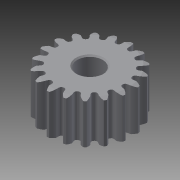
# Autodesk Inventor part: GEAHB1.0-18-10-A-6_b
Saved by Autodesk Inventor 2014 SP2 (Build 180246200, 246)
## iProperties
Created: 2019-03-13
Part Number: GEAHB1.0-18-10-A-6_b
Material: Generic
Catalog Web Link: www.cadenas.de
Description: GEAHB1.0, GEAHBB1.0, GEAHBG1.0, GEAHS1.0, GEAB1.0, GEABB1.0, GEABG1.0, GEAS1.0, GEAKB1.0, GEAKBB1.0, GEAKBG1.0, GEAKS1.0_body-Spur Gears - Pressure Angle 20 Degree Module 1.0
Vendor: MISUMI
Document SubType Name: Modeling
Designer: psadmin
Manufacturer: MISUMI
Mass: 2.186 g
Surface Area: 17.0541 cm^2
Volume: 2.186 cm^3
Density: 1 g/cm^3
Appearance: PSOLRGB-192-192-192
Category: PARTsolutions
Company: MISUMI
Title: GEAHB1.0-18-10-A-6
Author: Cadenas PARTsolutions
Comments: Spur Gears - Pressure Angle 20 Degree Module 1.0
PSOL_IDENT_0: {$CADENAS_DATA\23d-libs\misumi\metric\54_spur_gears\geab10\geab10.prj},526 {VTYP=3D},{NB=GEAHB1.0-18
PSOL_IDENT_1: -10-A-6_b},{LINA=GEAHB1.0-18-10-A-6},{NN=GEAHB1.0, GEAHBB1.0, GEAHBG1.0, GEAHS1.0, GEAB1.0, GEABB1.0
PSOL_IDENT_2: , GEABG1.0, GEAS1.0, GEAKB1.0, GEAKBB1.0, GEAKBG1.0, GEAKS1.0_body},{DATE=12.06.2018 01:08:09},{GEOM
PSOL_IDENT_3: DATE=12.06.2018 01:08:00},{VERSION=},{LINEID=20},{WBVAR=SHS,MAT,ST,NT,B,TSSE,TS,PS,ALT1,ALT2,TPC,ALT
PSOL_IDENT_4: 11,ALT10,BS,ALT4,Z,J,ALT5,Q,R,S,T,ALT9,SRG,ALT6,LFC,LTC,MALT6,ALT7,KFC,KTC,K,ALT3,DIRALT3,QFC,QTC,MA
PSOL_IDENT_5: LT3,ALT8,DIRALT8,ZFC,ZTC,U},{WBNUMERIC=NT,B,BS,Z,J,Q,R,S,T,SRG,LFC,LTC,KFC,KTC,K,QFC,QTC,ZFC,ZTC,U}
PSOL_IDENT_6: {NB=GEAHB1.0-18-10-A-6_b},{LINA=GEAHB1.0-18-10-A-6},{KT=DUMMY},{PN=GEAHB1.0-18-10-A-6},{SHS=RH},{TY
PSOL_IDENT_7: PE=GEAHB},{MAT=S45C},{MATALG= 'S45C','S45C Equivalent','SUS304','SUS304' },{ST=},{STALG= '','-','BO'
PSOL_IDENT_8: ,'Black Oxide','ENP','Electroless Nickel Plating'},{AC=-},{MOD=1.0},{NT=18},{NTALG=12,13,14,15,16,17
PSOL_IDENT_9: ,18,19,20,21,22,23,24,25,26,27,28,29,30,32,33,34,35,36,38,39,40,42,44,45,46,48,49,50,51,52,54,55,56,
PSOL_IDENT_10: 57,58,60,62,63,64,65,66,68,69,70,72,75,76,77,78,80,81,84,85,88,90,91,92,95,96,98,99,100,110,120},{B=
PSOL_IDENT_11: 10},{BALG=6,8,10,12},{TSSE=TSSE},{TSSEALG= '','Not Specified','TSSE','Specified'},{TS=A},{TSALG='K','
PSOL_IDENT_12: K','A','A'},{TSPN=-A},{PS=6},{PSALG='6','6','6.35','6.35','7','7','8','8','9','9','10','10','11','11'
PSOL_IDENT_13: ,'12','12'},{P=6.00},{DD=18},{D=20},{G=15.5},{H=0},{L=0},{LL1=0},{LL2=0},{M=-},{ML=0.000},{ALT1=},{A
PSOL_IDENT_14: LT1ALG= '','N/A' },{ALT1PN=},{KC=0},{ALT2=},{ALT2ALG= '','N/A' },{TPC=N/A},{TPCALG= 'N/A' },{ALT2PN=
PSOL_IDENT_15: },{ALT11=},{ALT11ALG= '','N/A' },{ALT11PN=},{DEG=0},{ALT10=},{ALT10ALG= '','Not applicable' },{BS=0.
PSOL_IDENT_16: 0},{BSALG=0},{BSMIN=3},{BSMAX=0},{ALT10PN=},{LL13D=0},{LL23D=0},{LBS=10},{ALT4=},{ALT4ALG='','w/o St
PSOL_IDENT_17: epped Hole','DHL','with DHL (Stepped Hole)','DHR','with DHR (Stepped Hole)'},{ALT41=1},{ALT42=1},{AL
PSOL_IDENT_18: T4PN=},{Z=0},{ZALG=0},{ZPN=},{ZMINL=8},{ZMAXL=11},{ZMINR=8},{ZMAXR=11},{J=0.0},{JALG=0},{JPN=},{JMIN=
PSOL_IDENT_19: 2.0},{JMAX=0.0},{ALT5=},{ALT5ALG= '','w/o WDH (Both Ends Stepped Hole)','WDH','with WDH (Both Ends S
PSOL_IDENT_20: tepped Hole)' },{ALT5PN=},{Q=0},{QALG=0},{QPN=},{QMIN=8},{QMAX=11},{R=0},{RALG=0},{RPN=},{RMIN=8},{R
PSOL_IDENT_21: MAX=11.0},{S=0},{SALG=0},{SPN=},{SMIN=3},{SMAX=4},{T=0},{TALG=0},{TPN=},{TMIN=3},{TMAX=0},{ALT9=},{A
PSOL_IDENT_22: LT9ALG= '','Not applicable' },{SRG=0.0},{SRGALG=0},{SRGMIN=3.500},{SRGMINALG=3.500},{SRGMAX=0.000},{
PSOL_IDENT_23: SRGMAXALG=0.000},{DD2=0.0},{MM=0.00},{NN=0.00},{DD2ALG=0.000},{MMALG=0.000},{NNALG=0.000},{ALT9PN=},
PSOL_IDENT_24: {ALT6=},{ALT6ALG= '','Not applicable' },{ALT6PN=},{LFC=0},{LFCALG=0},{LTC=0},{LTCALG=0},{LPCDMIN=14}
PSOL_IDENT_25: ,{LPCDMAX=8},{MALT6=N/A},{MALT6ALG= 'N/A' },{C=0.0},{ALT7=},{ALT7ALG= '','Not applicable' },{ALT7PN=
PSOL_IDENT_26: },{KFC=0},{KFCALG=[0]},{KTC=0},{KTCALG=[0]},{KPCDMIN1=13},{KPCDMAX1=-7},{KPCDMIN2=7},{KPCDMAX2=8},{K
PSOL_IDENT_27: PCD=0},{K=0.0},{KALG=[0]},{KALT7L=10},{SCREW=0},{SCREWL=0},{ALT3=},{ALT3ALG= '','Not applicable' },{
PSOL_IDENT_28: DIRALT3=},{DIRALT3ALG= '','N/A' },{ALT3PN=},{QFC=0},{QFCALG=[0]},{QTC=0},{QTCALG=[0]},{QPCDMIN1=13},
PSOL_IDENT_29: {QPCDMAX1=-7},{QPCDMIN2=7},{QPCDMAX2=8},{CIFMALT3=3},{QPCD=0},{MALT3=N/A},{MALT3ALG= 'N/A' },{MALT3L=
PSOL_IDENT_30: 0},{MS1=3},{PITCH=0},{BB=0},{TT=0},{ALT8=},{ALT8ALG= '','Not applicable' },{DIRALT8=},{DIRALT8ALG= ''
PSOL_IDENT_31: ,'N/A' },{ALT8PN=},{ZFC=0},{ZFCALG=[0]},{ZFCMIN=16},{ZFCMAX=5},{ZTC=0},{ZTCALG=[0]},{ZPCDMIN1=16},{Z
PSOL_IDENT_32: PCDMIN2=11},{ZPCDMAX1=-10},{ZPCDMAX2=5},{ZPCD=0},{U=0},{UALG=[0]},{UMAX=0},{UMAX1=0},{UMAX2=4},{UMIN=
PSOL_IDENT_33: 3},{U1=0.0},{U2=0.0},{F=0.0},{PLANE=3},{BL1=10},{BL2=9.5},{PCD=0},{SHN=0},{SHDEG1=0},{SHDEG2=0},{PZQ
PSOL_IDENT_34: RDD2=6},{ALT3LBS=9.5},{D1=5},{D2=10},{D3=20},{D4=0.1},{D5=3},{D6=2.769231},{D7=0.85},{D8=0.5},{D9=0.
PSOL_IDENT_35: 812072},{S1=15},{S2=1},{KR=22.5}
NN: 0
NT: 18
NB: GEAHB1.0-18-10-A-6_b
NBSYN: $PN._b
LINA: GEAHB1.0-18-10-A-6
PN: GEAHB1.0-18-10-A-6
SHS: Round Hole
MAT: S45C Equivalent
ST: -
AC: -
MOD: 1
B: 10
TSSE: Specified
TS: A
PS: 6
DD: 18
D: 20
G: 15.5
H: 0
L: 0
LL1: 0
LL2: 0
M: -
ALT1: N/A
ALT2: N/A
TPC: N/A
ALT11: N/A
ALT10: Not applicable
BS: 0
ALT4: w/o Stepped Hole
Z: 0
J: 0
ALT5: w/o WDH (Both Ends Stepped Hole)
Q: 0
R: 0
S: 0
T: 0
ALT9: Not applicable
SRG: 0
DD2: 0
MM: 0
ALT6: Not applicable
LFC: 0
LTC: 0
MALT6: N/A
C: 0
ALT7: Not applicable
KFC: 0
KTC: 0
K: 0
ALT3: Not applicable
DIRALT3: N/A
QFC: 0
QTC: 0
MALT3: N/A
ALT8: Not applicable
DIRALT8: N/A
ZFC: 0
ZTC: 0
U: 0
U1: 0
U2: 0
F: 0
SUPPLIER: MISUMI
ARTICLENO: GEAHB1.0-18-10-A-6_b
BOMINFO: GEAHB1.0-18-10-A-6
CREATOR: CADENAS GmbH
Autodesk Inventor part; units mm, degrees
sketch "Sketch_12" plane through (0, 0, 0) normal (1, 0, 0) x (0, 1, 0)
  line L0 (0, 0) -> (0, 10)
  line L1 (0, 10) -> (9, 10)
  line L2 (9, 10) -> (15, 8.3923)
  line L3 (15, 8.3923) -> (15, 1.6077)
  line L4 (15, 1.6077) -> (9, 0)
  line L5 (9, 0) -> (0, 0)
  line L6 (0, 0) -> (0, 10)
  constraints: 14 end point
revolve "Revolution1" add sketch "Sketch_12" angle 360 about axis through (0, 0, 0) along (0, 0, -1)
sketch "Sketch_3" plane through (0, 0, 0) normal (0, 0, 1) x (1, 0, 0)
  circle A0 centre (0, 0) radius 40
  arc A1 (-9.8858, 1.507) -> (-9.859, 1.4225) centre (-9.7869, 1.4919) ccw
  arc A2 (-9.859, 1.4225) -> (-8.9658, 0.7844) centre (-7.6979, 3.5033) ccw
  arc A3 (-8.9658, 0.7844) -> (-8.707, 0.7127) centre (-8.6226, 1.5204) ccw
  arc A4 (-8.0844, 0.573) -> (-8.707, 0.7127) centre (-8.9979, -2.0412) ccw
  arc A5 (-7.7494, 0.0949) -> (-8.0844, 0.573) centre (-8.2494, 0.101) ccw
  arc A6 (-7.7494, 0.0949) -> (-7.7494, -0.0949) centre (0, 0) ccw
  arc A7 (-8.0844, -0.573) -> (-7.7494, -0.0949) centre (-8.2494, -0.101) ccw
  arc A8 (-8.707, -0.7127) -> (-8.0844, -0.573) centre (-8.9979, 2.0412) ccw
  arc A9 (-8.707, -0.7127) -> (-8.9658, -0.7844) centre (-8.6226, -1.5204) ccw
  arc A10 (-8.9658, -0.7844) -> (-9.859, -1.4225) centre (-7.6979, -3.5033) ccw
  arc A11 (-9.859, -1.4225) -> (-9.8858, -1.507) centre (-9.7869, -1.4919) ccw
  arc A12 (-9.8858, -1.507) -> (-9.805, -1.9651) centre (0, 0) ccw
  arc A13 (-9.805, -1.9651) -> (-9.7509, -2.0352) centre (-9.707, -1.9454) ccw
  arc A14 (-9.7509, -2.0352) -> (-8.6933, -2.3294) centre (-8.4319, 0.6592) ccw
  arc A15 (-8.6933, -2.3294) -> (-8.4257, -2.3082) centre (-8.6226, -1.5204) ccw
  arc A16 (-7.7929, -2.2266) -> (-8.4257, -2.3082) centre (-7.7572, -4.9956) ccw
  arc A17 (-7.3145, -2.5613) -> (-7.7929, -2.2266) centre (-7.7864, -2.7265) ccw
  arc A18 (-7.3145, -2.5613) -> (-7.2496, -2.7396) centre (0, 0) ccw
  arc A19 (-7.4009, -3.3035) -> (-7.2496, -2.7396) centre (-7.7173, -2.9164) ccw
  arc A20 (-7.9381, -3.6477) -> (-7.4009, -3.3035) centre (-9.1534, -1.1594) ccw
  arc A21 (-7.9381, -3.6477) -> (-8.1568, -3.8036) centre (-7.5825, -4.3778) ccw
  arc A22 (-8.1568, -3.8036) -> (-8.7779, -4.7087) centre (-6.0354, -5.9249) ccw
  arc A23 (-8.7779, -4.7087) -> (-8.7742, -4.7972) centre (-8.6865, -4.7492) ccw
  arc A24 (-8.7742, -4.7972) -> (-8.5416, -5.2001) centre (0, 0) ccw
  arc A25 (-8.5416, -5.2001) -> (-8.4668, -5.2475) centre (-8.4562, -5.1481) ccw
  arc A26 (-8.4668, -5.2475) -> (-7.3724, -5.1622) centre (-8.1488, -2.2644) ccw
  arc A27 (-7.3724, -5.1622) -> (-7.1281, -5.0508) centre (-7.5825, -4.3778) ccw
  arc A28 (-6.5614, -4.7576) -> (-7.1281, -5.0508) centre (-5.5808, -7.3474) ccw
  arc A29 (-5.9974, -4.9085) -> (-6.5614, -4.7576) centre (-6.3843, -5.2252) ccw
  arc A30 (-5.9974, -4.9085) -> (-5.8754, -5.0539) centre (0, 0) ccw
  arc A31 (-5.8247, -5.6356) -> (-5.8754, -5.0539) centre (-6.2545, -5.38) ccw
  arc A32 (-6.2118, -6.1427) -> (-5.8247, -5.6356) centre (-8.2049, -4.2201) ccw
  arc A33 (-6.2118, -6.1427) -> (-6.364, -6.364) centre (-5.628, -6.7072) ccw
  arc A34 (-6.364, -6.364) -> (-6.638, -7.4269) centre (-3.645, -7.6318) ccw
  arc A35 (-6.638, -7.4269) -> (-6.6043, -7.5089) centre (-6.5383, -7.4338) ccw
  arc A36 (-6.6043, -7.5089) -> (-6.248, -7.8079) centre (0, 0) ccw
  arc A37 (-6.248, -7.8079) -> (-6.1614, -7.8269) centre (-6.1855, -7.7298) ccw
  arc A38 (-6.1614, -7.8269) -> (-5.1622, -7.3724) centre (-6.8829, -4.9149) ccw
  arc A39 (-5.1622, -7.3724) -> (-4.9707, -7.1841) centre (-5.628, -6.7072) ccw
  arc A40 (-4.5385, -6.7148) -> (-4.9707, -7.1841) centre (-2.7312, -8.813) ccw
  arc A41 (-3.9569, -6.6637) -> (-4.5385, -6.7148) centre (-4.2122, -7.0937) ccw
  arc A42 (-3.9569, -6.6637) -> (-3.7925, -6.7586) centre (0, 0) ccw
  arc A43 (-3.546, -7.2879) -> (-3.7925, -6.7586) centre (-4.0372, -7.1947) ccw
  arc A44 (-3.7363, -7.8968) -> (-3.546, -7.2879) centre (-6.2667, -6.7718) ccw
  arc A45 (-3.7363, -7.8968) -> (-3.8036, -8.1568) centre (-2.9946, -8.2275) ccw
  arc A46 (-3.8036, -8.1568) -> (-3.6975, -9.2494) centre (-0.815, -8.4182) ccw
  arc A47 (-3.6975, -9.2494) -> (-3.6378, -9.3148) centre (-3.6015, -9.2217) ccw
  arc A48 (-3.6378, -9.3148) -> (-3.2007, -9.4739) centre (0, 0) ccw
  arc A49 (-3.2007, -9.4739) -> (-3.1129, -9.4622) centre (-3.1687, -9.3792) ccw
  arc A50 (-3.1129, -9.4622) -> (-2.3294, -8.6933) centre (-4.7868, -6.9726) ccw
  arc A51 (-2.3294, -8.6933) -> (-2.2138, -8.4509) centre (-2.9946, -8.2275) ccw
  arc A52 (-1.9682, -7.8621) -> (-2.2138, -8.4509) centre (0.4477, -9.2157) ccw
  arc A53 (-1.4391, -7.6152) -> (-1.9682, -7.8621) centre (-1.532, -8.1065) ccw
  arc A54 (-1.4391, -7.6152) -> (-1.2522, -7.6482) centre (0, 0) ccw
  arc A55 (-0.8395, -8.0611) -> (-1.2522, -7.6482) centre (-1.333, -8.1416) ccw
  arc A56 (-0.8101, -8.6985) -> (-0.8395, -8.0611) centre (-3.5727, -8.5068) ccw
  arc A57 (-0.8101, -8.6985) -> (-0.7844, -8.9658) centre (0, -8.7556) ccw
  arc A58 (-0.7844, -8.9658) -> (-0.3111, -9.9562) centre (2.1134, -8.1893) ccw
  arc A59 (-0.3111, -9.9562) -> (-0.2326, -9.9973) centre (-0.2303, -9.8973) ccw
  arc A60 (-0.2326, -9.9973) -> (0.2326, -9.9973) centre (0, 0) ccw
  arc A61 (0.2326, -9.9973) -> (0.3111, -9.9562) centre (0.2303, -9.8973) ccw
  arc A62 (0.3111, -9.9562) -> (0.7844, -8.9658) centre (-2.1134, -8.1893) ccw
  arc A63 (0.7844, -8.9658) -> (0.8101, -8.6985) centre (0, -8.7556) ccw
  arc A64 (0.8395, -8.0611) -> (0.8101, -8.6985) centre (3.5727, -8.5068) ccw
  arc A65 (1.2522, -7.6482) -> (0.8395, -8.0611) centre (1.333, -8.1416) ccw
  arc A66 (1.2522, -7.6482) -> (1.4391, -7.6152) centre (0, 0) ccw
  arc A67 (1.9682, -7.8621) -> (1.4391, -7.6152) centre (1.532, -8.1065) ccw
  arc A68 (2.2138, -8.4509) -> (1.9682, -7.8621) centre (-0.4477, -9.2157) ccw
  arc A69 (2.2138, -8.4509) -> (2.3294, -8.6933) centre (2.9946, -8.2275) ccw
  arc A70 (2.3294, -8.6933) -> (3.1129, -9.4622) centre (4.7868, -6.9726) ccw
  arc A71 (3.1129, -9.4622) -> (3.2007, -9.4739) centre (3.1687, -9.3792) ccw
  arc A72 (3.2007, -9.4739) -> (3.6378, -9.3148) centre (0, 0) ccw
  arc A73 (3.6378, -9.3148) -> (3.6975, -9.2494) centre (3.6015, -9.2217) ccw
  arc A74 (3.6975, -9.2494) -> (3.8036, -8.1568) centre (0.815, -8.4182) ccw
  arc A75 (3.8036, -8.1568) -> (3.7363, -7.8968) centre (2.9946, -8.2275) ccw
  arc A76 (3.546, -7.2879) -> (3.7363, -7.8968) centre (6.2667, -6.7718) ccw
  arc A77 (3.7925, -6.7586) -> (3.546, -7.2879) centre (4.0372, -7.1947) ccw
  arc A78 (3.7925, -6.7586) -> (3.9569, -6.6637) centre (0, 0) ccw
  arc A79 (4.5385, -6.7148) -> (3.9569, -6.6637) centre (4.2122, -7.0937) ccw
  arc A80 (4.9707, -7.1841) -> (4.5385, -6.7148) centre (2.7312, -8.813) ccw
  arc A81 (4.9707, -7.1841) -> (5.1622, -7.3724) centre (5.628, -6.7072) ccw
  arc A82 (5.1622, -7.3724) -> (6.1614, -7.8269) centre (6.8829, -4.9149) ccw
  arc A83 (6.1614, -7.8269) -> (6.248, -7.8079) centre (6.1855, -7.7298) ccw
  arc A84 (6.248, -7.8079) -> (6.6043, -7.5089) centre (0, 0) ccw
  arc A85 (6.6043, -7.5089) -> (6.638, -7.4269) centre (6.5383, -7.4338) ccw
  arc A86 (6.638, -7.4269) -> (6.364, -6.364) centre (3.645, -7.6318) ccw
  arc A87 (6.364, -6.364) -> (6.2118, -6.1427) centre (5.628, -6.7072) ccw
  arc A88 (5.8247, -5.6356) -> (6.2118, -6.1427) centre (8.2049, -4.2201) ccw
  arc A89 (5.8754, -5.0539) -> (5.8247, -5.6356) centre (6.2545, -5.38) ccw
  arc A90 (5.8754, -5.0539) -> (5.9974, -4.9085) centre (0, 0) ccw
  arc A91 (6.5614, -4.7576) -> (5.9974, -4.9085) centre (6.3843, -5.2252) ccw
  arc A92 (7.1281, -5.0508) -> (6.5614, -4.7576) centre (5.5808, -7.3474) ccw
  arc A93 (7.1281, -5.0508) -> (7.3724, -5.1622) centre (7.5825, -4.3778) ccw
  arc A94 (7.3724, -5.1622) -> (8.4668, -5.2475) centre (8.1488, -2.2644) ccw
  arc A95 (8.4668, -5.2475) -> (8.5416, -5.2001) centre (8.4562, -5.1481) ccw
  arc A96 (8.5416, -5.2001) -> (8.7742, -4.7972) centre (0, 0) ccw
  arc A97 (8.7742, -4.7972) -> (8.7779, -4.7087) centre (8.6865, -4.7492) ccw
  arc A98 (8.7779, -4.7087) -> (8.1568, -3.8036) centre (6.0354, -5.9249) ccw
  arc A99 (8.1568, -3.8036) -> (7.9381, -3.6477) centre (7.5825, -4.3778) ccw
  arc A100 (7.4009, -3.3035) -> (7.9381, -3.6477) centre (9.1534, -1.1594) ccw
  arc A101 (7.2496, -2.7396) -> (7.4009, -3.3035) centre (7.7173, -2.9164) ccw
  arc A102 (7.2496, -2.7396) -> (7.3145, -2.5613) centre (0, 0) ccw
  arc A103 (7.7929, -2.2266) -> (7.3145, -2.5613) centre (7.7864, -2.7265) ccw
  arc A104 (8.4257, -2.3082) -> (7.7929, -2.2266) centre (7.7572, -4.9956) ccw
  arc A105 (8.4257, -2.3082) -> (8.6933, -2.3294) centre (8.6226, -1.5204) ccw
  arc A106 (8.6933, -2.3294) -> (9.7509, -2.0352) centre (8.4319, 0.6592) ccw
  arc A107 (9.7509, -2.0352) -> (9.805, -1.9651) centre (9.707, -1.9454) ccw
  arc A108 (9.805, -1.9651) -> (9.8858, -1.507) centre (0, 0) ccw
  arc A109 (9.8858, -1.507) -> (9.859, -1.4225) centre (9.7869, -1.4919) ccw
  arc A110 (9.859, -1.4225) -> (8.9658, -0.7844) centre (7.6979, -3.5033) ccw
  arc A111 (8.9658, -0.7844) -> (8.707, -0.7127) centre (8.6226, -1.5204) ccw
  arc A112 (8.0844, -0.573) -> (8.707, -0.7127) centre (8.9979, 2.0412) ccw
  arc A113 (7.7494, -0.0949) -> (8.0844, -0.573) centre (8.2494, -0.101) ccw
  arc A114 (7.7494, -0.0949) -> (7.7494, 0.0949) centre (0, 0) ccw
  arc A115 (8.0844, 0.573) -> (7.7494, 0.0949) centre (8.2494, 0.101) ccw
  arc A116 (8.707, 0.7127) -> (8.0844, 0.573) centre (8.9979, -2.0412) ccw
  arc A117 (8.707, 0.7127) -> (8.9658, 0.7844) centre (8.6226, 1.5204) ccw
  arc A118 (8.9658, 0.7844) -> (9.859, 1.4225) centre (7.6979, 3.5033) ccw
  arc A119 (9.859, 1.4225) -> (9.8858, 1.507) centre (9.7869, 1.4919) ccw
  arc A120 (9.8858, 1.507) -> (9.805, 1.9651) centre (0, 0) ccw
  arc A121 (9.805, 1.9651) -> (9.7509, 2.0352) centre (9.707, 1.9454) ccw
  arc A122 (9.7509, 2.0352) -> (8.6933, 2.3294) centre (8.4319, -0.6592) ccw
  arc A123 (8.6933, 2.3294) -> (8.4257, 2.3082) centre (8.6226, 1.5204) ccw
  arc A124 (7.7929, 2.2266) -> (8.4257, 2.3082) centre (7.7572, 4.9956) ccw
  arc A125 (7.3145, 2.5613) -> (7.7929, 2.2266) centre (7.7864, 2.7265) ccw
  arc A126 (7.3145, 2.5613) -> (7.2496, 2.7396) centre (0, 0) ccw
  arc A127 (7.4009, 3.3035) -> (7.2496, 2.7396) centre (7.7173, 2.9164) ccw
  arc A128 (7.9381, 3.6477) -> (7.4009, 3.3035) centre (9.1534, 1.1594) ccw
  arc A129 (7.9381, 3.6477) -> (8.1568, 3.8036) centre (7.5825, 4.3778) ccw
  arc A130 (8.1568, 3.8036) -> (8.7779, 4.7087) centre (6.0354, 5.9249) ccw
  arc A131 (8.7779, 4.7087) -> (8.7742, 4.7972) centre (8.6865, 4.7492) ccw
  arc A132 (8.7742, 4.7972) -> (8.5416, 5.2001) centre (0, 0) ccw
  arc A133 (8.5416, 5.2001) -> (8.4668, 5.2475) centre (8.4562, 5.1481) ccw
  arc A134 (8.4668, 5.2475) -> (7.3724, 5.1622) centre (8.1488, 2.2644) ccw
  arc A135 (7.3724, 5.1622) -> (7.1281, 5.0508) centre (7.5825, 4.3778) ccw
  arc A136 (6.5614, 4.7576) -> (7.1281, 5.0508) centre (5.5808, 7.3474) ccw
  arc A137 (5.9974, 4.9085) -> (6.5614, 4.7576) centre (6.3843, 5.2252) ccw
  arc A138 (5.9974, 4.9085) -> (5.8754, 5.0539) centre (0, 0) ccw
  arc A139 (5.8247, 5.6356) -> (5.8754, 5.0539) centre (6.2545, 5.38) ccw
  arc A140 (6.2118, 6.1427) -> (5.8247, 5.6356) centre (8.2049, 4.2201) ccw
  arc A141 (6.2118, 6.1427) -> (6.364, 6.364) centre (5.628, 6.7072) ccw
  arc A142 (6.364, 6.364) -> (6.638, 7.4269) centre (3.645, 7.6318) ccw
  arc A143 (6.638, 7.4269) -> (6.6043, 7.5089) centre (6.5383, 7.4338) ccw
  arc A144 (6.6043, 7.5089) -> (6.248, 7.8079) centre (0, 0) ccw
  arc A145 (6.248, 7.8079) -> (6.1614, 7.8269) centre (6.1855, 7.7298) ccw
  arc A146 (6.1614, 7.8269) -> (5.1622, 7.3724) centre (6.8829, 4.9149) ccw
  arc A147 (5.1622, 7.3724) -> (4.9707, 7.1841) centre (5.628, 6.7072) ccw
  arc A148 (4.5385, 6.7148) -> (4.9707, 7.1841) centre (2.7312, 8.813) ccw
  arc A149 (3.9569, 6.6637) -> (4.5385, 6.7148) centre (4.2122, 7.0937) ccw
  arc A150 (3.9569, 6.6637) -> (3.7925, 6.7586) centre (0, 0) ccw
  arc A151 (3.546, 7.2879) -> (3.7925, 6.7586) centre (4.0372, 7.1947) ccw
  arc A152 (3.7363, 7.8968) -> (3.546, 7.2879) centre (6.2667, 6.7718) ccw
  arc A153 (3.7363, 7.8968) -> (3.8036, 8.1568) centre (2.9946, 8.2275) ccw
  arc A154 (3.8036, 8.1568) -> (3.6975, 9.2494) centre (0.815, 8.4182) ccw
  arc A155 (3.6975, 9.2494) -> (3.6378, 9.3148) centre (3.6015, 9.2217) ccw
  arc A156 (3.6378, 9.3148) -> (3.2007, 9.4739) centre (0, 0) ccw
  arc A157 (3.2007, 9.4739) -> (3.1129, 9.4622) centre (3.1687, 9.3792) ccw
  arc A158 (3.1129, 9.4622) -> (2.3294, 8.6933) centre (4.7868, 6.9726) ccw
  arc A159 (2.3294, 8.6933) -> (2.2138, 8.4509) centre (2.9946, 8.2275) ccw
  arc A160 (1.9682, 7.8621) -> (2.2138, 8.4509) centre (-0.4477, 9.2157) ccw
  arc A161 (1.4391, 7.6152) -> (1.9682, 7.8621) centre (1.532, 8.1065) ccw
  arc A162 (1.4391, 7.6152) -> (1.2522, 7.6482) centre (0, 0) ccw
  arc A163 (0.8395, 8.0611) -> (1.2522, 7.6482) centre (1.333, 8.1416) ccw
  arc A164 (0.8101, 8.6985) -> (0.8395, 8.0611) centre (3.5727, 8.5068) ccw
  arc A165 (0.8101, 8.6985) -> (0.7844, 8.9658) centre (0, 8.7556) ccw
  arc A166 (0.7844, 8.9658) -> (0.3111, 9.9562) centre (-2.1134, 8.1893) ccw
  arc A167 (0.3111, 9.9562) -> (0.2326, 9.9973) centre (0.2303, 9.8973) ccw
  arc A168 (0.2326, 9.9973) -> (-0.2326, 9.9973) centre (0, 0) ccw
  arc A169 (-0.2326, 9.9973) -> (-0.3111, 9.9562) centre (-0.2303, 9.8973) ccw
  arc A170 (-0.3111, 9.9562) -> (-0.7844, 8.9658) centre (2.1134, 8.1893) ccw
  arc A171 (-0.7844, 8.9658) -> (-0.8101, 8.6985) centre (0, 8.7556) ccw
  arc A172 (-0.8395, 8.0611) -> (-0.8101, 8.6985) centre (-3.5727, 8.5068) ccw
  arc A173 (-1.2522, 7.6482) -> (-0.8395, 8.0611) centre (-1.333, 8.1416) ccw
  arc A174 (-1.2522, 7.6482) -> (-1.4391, 7.6152) centre (0, 0) ccw
  arc A175 (-1.9682, 7.8621) -> (-1.4391, 7.6152) centre (-1.532, 8.1065) ccw
  arc A176 (-2.2138, 8.4509) -> (-1.9682, 7.8621) centre (0.4477, 9.2157) ccw
  arc A177 (-2.2138, 8.4509) -> (-2.3294, 8.6933) centre (-2.9946, 8.2275) ccw
  arc A178 (-2.3294, 8.6933) -> (-3.1129, 9.4622) centre (-4.7868, 6.9726) ccw
  arc A179 (-3.1129, 9.4622) -> (-3.2007, 9.4739) centre (-3.1687, 9.3792) ccw
  arc A180 (-3.2007, 9.4739) -> (-3.6378, 9.3148) centre (0, 0) ccw
  arc A181 (-3.6378, 9.3148) -> (-3.6975, 9.2494) centre (-3.6015, 9.2217) ccw
  arc A182 (-3.6975, 9.2494) -> (-3.8036, 8.1568) centre (-0.815, 8.4182) ccw
  arc A183 (-3.8036, 8.1568) -> (-3.7363, 7.8968) centre (-2.9946, 8.2275) ccw
  arc A184 (-3.546, 7.2879) -> (-3.7363, 7.8968) centre (-6.2667, 6.7718) ccw
  arc A185 (-3.7925, 6.7586) -> (-3.546, 7.2879) centre (-4.0372, 7.1947) ccw
  arc A186 (-3.7925, 6.7586) -> (-3.9569, 6.6637) centre (0, 0) ccw
  arc A187 (-4.5385, 6.7148) -> (-3.9569, 6.6637) centre (-4.2122, 7.0937) ccw
  arc A188 (-4.9707, 7.1841) -> (-4.5385, 6.7148) centre (-2.7312, 8.813) ccw
  arc A189 (-4.9707, 7.1841) -> (-5.1622, 7.3724) centre (-5.628, 6.7072) ccw
  arc A190 (-5.1622, 7.3724) -> (-6.1614, 7.8269) centre (-6.8829, 4.9149) ccw
  arc A191 (-6.1614, 7.8269) -> (-6.248, 7.8079) centre (-6.1855, 7.7298) ccw
  arc A192 (-6.248, 7.8079) -> (-6.6043, 7.5089) centre (0, 0) ccw
  arc A193 (-6.6043, 7.5089) -> (-6.638, 7.4269) centre (-6.5383, 7.4338) ccw
  arc A194 (-6.638, 7.4269) -> (-6.364, 6.364) centre (-3.645, 7.6318) ccw
  arc A195 (-6.364, 6.364) -> (-6.2118, 6.1427) centre (-5.628, 6.7072) ccw
  arc A196 (-5.8247, 5.6356) -> (-6.2118, 6.1427) centre (-8.2049, 4.2201) ccw
  arc A197 (-5.8754, 5.0539) -> (-5.8247, 5.6356) centre (-6.2545, 5.38) ccw
  arc A198 (-5.8754, 5.0539) -> (-5.9974, 4.9085) centre (0, 0) ccw
  arc A199 (-6.5614, 4.7576) -> (-5.9974, 4.9085) centre (-6.3843, 5.2252) ccw
  arc A200 (-7.1281, 5.0508) -> (-6.5614, 4.7576) centre (-5.5808, 7.3474) ccw
  arc A201 (-7.1281, 5.0508) -> (-7.3724, 5.1622) centre (-7.5825, 4.3778) ccw
  arc A202 (-7.3724, 5.1622) -> (-8.4668, 5.2475) centre (-8.1488, 2.2644) ccw
  arc A203 (-8.4668, 5.2475) -> (-8.5416, 5.2001) centre (-8.4562, 5.1481) ccw
  arc A204 (-8.5416, 5.2001) -> (-8.7742, 4.7972) centre (0, 0) ccw
  arc A205 (-8.7742, 4.7972) -> (-8.7779, 4.7087) centre (-8.6865, 4.7492) ccw
  arc A206 (-8.7779, 4.7087) -> (-8.1568, 3.8036) centre (-6.0354, 5.9249) ccw
  arc A207 (-8.1568, 3.8036) -> (-7.9381, 3.6477) centre (-7.5825, 4.3778) ccw
  arc A208 (-7.4009, 3.3035) -> (-7.9381, 3.6477) centre (-9.1534, 1.1594) ccw
  arc A209 (-7.2496, 2.7396) -> (-7.4009, 3.3035) centre (-7.7173, 2.9164) ccw
  arc A210 (-7.2496, 2.7396) -> (-7.3145, 2.5613) centre (0, 0) ccw
  arc A211 (-7.7929, 2.2266) -> (-7.3145, 2.5613) centre (-7.7864, 2.7265) ccw
  arc A212 (-8.4257, 2.3082) -> (-7.7929, 2.2266) centre (-7.7572, 4.9956) ccw
  arc A213 (-8.4257, 2.3082) -> (-8.6933, 2.3294) centre (-8.6226, 1.5204) ccw
  arc A214 (-8.6933, 2.3294) -> (-9.7509, 2.0352) centre (-8.4319, -0.6592) ccw
  arc A215 (-9.7509, 2.0352) -> (-9.805, 1.9651) centre (-9.707, 1.9454) ccw
  arc A216 (-9.805, 1.9651) -> (-9.8858, 1.507) centre (0, 0) ccw
  constraints: 432 point on circle, 217 centre point
extrude "Extrusion1" cut sketch "Sketch_3" along normal blind 11
sketch "Sketch3" plane through (0, 0, 0) normal (0, 0, -1) x (-1, 0, 0)
  point P0 (0, 0)
hole "Hole1" at (0, 0, 0) direction (0, 0, 1) diameter 6 depth 10
sketch "_____7" plane through (0, 0, 0) normal (1, 0, 0) x (0, 0, -1)
  line L0 (500, 0) -> (-500, 0)
  line L1 (-0.3, 3) -> (0, 3)
  line L2 (0, 3) -> (0, 3.3)
  line L3 (0, 3.3) -> (-0.3, 3)
  constraints: 8 end point
revolve "Revolution2" cut sketch "_____7" angle 360 about axis through (0, 0, -500) along (0, 0, -1)
sketch "_____17" plane through (0, 0, 0) normal (1, 0, 0) x (0, 0, -1)
  line L0 (500, 0) -> (-500, 0)
  line L1 (-10, 3.3) -> (-10, 3)
  line L2 (-10, 3) -> (-9.7, 3)
  line L3 (-9.7, 3) -> (-10, 3.3)
  constraints: 8 end point
revolve "Revolution3" cut sketch "_____17" angle 360 about axis through (0, 0, -500) along (0, 0, -1)
ref_plane "b_XY" through (0, 0, 0) normal (0, 0, 1) x (1, 0, 0)
ref_plane "b_YZ" through (0, 0, 0) normal (1, 0, 0) x (0, 1, 0)
ref_plane "b_ZX" through (0, 0, 0) normal (0, 1, 0) x (0, 0, 1)
ref_plane "turn_around_XY" through (0, 0, 0) normal (-1, 0, 0) x (0, 0, -1)
ref_plane "turn_around_YZ" through (0, 0, 0) normal (0, 0, -1) x (0, -1, 0)
ref_plane "turn_around_ZX" through (0, 0, 0) normal (0, -1, 0) x (-1, 0, 0)
body "Solid1"
